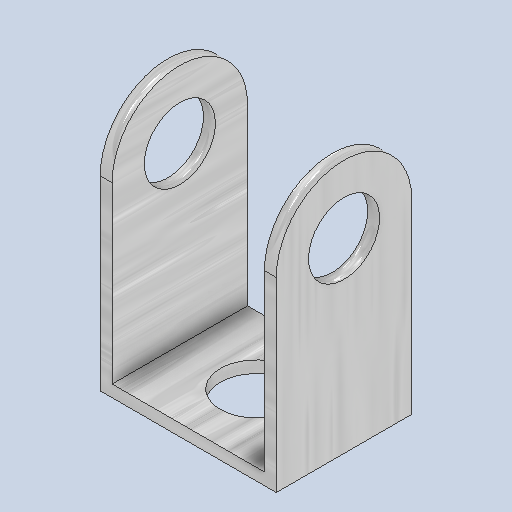
# Autodesk Inventor part: 각도엑추에이터브라켓
Saved by Autodesk Inventor 2024 (Build 280153000, 153)
## iProperties
Created: 2024-04-13
Part Number: 각도엑추에이터브라켓
Material: 스테인리스스틸
Document SubType Name: Modeling
Designer: kkamin5
Density: 8 g/cm^3
Appearance: 연마 브러시
Author: kkamin5
Autodesk Inventor part; units mm, degrees
ref_plane "YZ Plane" through (0, 0, 0) normal (1, 0, 0) x (0, 1, 0)
ref_plane "XZ Plane" through (0, 0, 0) normal (0, 1, 0) x (-1, 0, 0)
ref_plane "XY Plane" through (0, 0, 0) normal (0, 0, 1) x (1, 0, 0)
sketch "스케치1" plane through (0, 0, 0) normal (1, 0, 0) x (0, 1, 0)
  line L0 (-5.5, 4) -> (5.5, 4)
  line L1 (5.5, 4) -> (5.5, -4)
  line L2 (5.5, -4) -> (-5.5, -4)
  line L3 (-5.5, -4) -> (-5.5, 4)
  line L4 (-5.5, 4) -> (5.5, -4) construction
  line L5 (5.5, 4) -> (-5.5, -4) construction
  circle A0 centre (5.5, 0) radius 4
  circle A1 centre (5.5, 0) radius 2.1
  point P0 (0, 0)
  dimension "d0" = 8
  dimension "d1" = 11
  dimension "d2" = 4.2
  constraints: 12 end point, 3 midpoint, 2 parallel, 1 centre point, 1 coincident, 1 horizontal, 1 perpendicular, 3 other
  measures "d0" distance of L0.end L1.end
  measures "d1" distance of L1.end L2.end
  measures "d2" diameter of A1
extrude "돌출1" add sketch "스케치1" along normal mid plane 10.4 contours L0 A0 L2 L3 | A0 L1 A1 | L1 A1 A0
sketch "스케치2" plane through (-5.2, -5.5, 4) normal (0, 0, 1) x (1, 0, 0)
  line L0 (0.7, 17.0117) -> (9.7, 17.0117)
  line L1 (9.7, 17.0117) -> (9.7, 0.7)
  line L2 (9.7, 0.7) -> (0.7, 0.7)
  line L3 (0.7, 0.7) -> (0.7, 17.0117)
  line L4 (0.7, 17.0117) -> (9.7, 0.7) construction
  line L5 (9.7, 17.0117) -> (0.7, 0.7) construction
  line L6 (0, 0) -> (0, 11) projected
  line L7 (0, 0) -> (10.4, 0) projected
  line L8 (10.4, 11) -> (10.4, 0) projected
  point P0 (5.2, 5.5)
  point P1 (5.2, 8.8559)
  dimension "d5" = 0.7
  dimension "d6" = 0.7
  dimension "d7" = 0.7
  constraints: 12 end point, 2 midpoint, 2 parallel, 1 horizontal, 1 perpendicular
  measures "d5" distance between parallel lines of L6 L3
  measures "d6" distance between parallel lines of L7 L2
  measures "d7" distance between parallel lines of L8 L1
extrude "돌출2" cut sketch "스케치2" against normal through all
sketch "스케치3" plane through (-4.5, -4.8, 4) normal (0, 1, 0) x (1, 0, 0)
  circle A0 centre (4.5, 4) radius 2.1
  dimension "d10" = 4.2
  constraints: 1 centre point, 1 coincident
  measures "d10" diameter of A0
extrude "돌출3" cut sketch "스케치3" against normal through all
